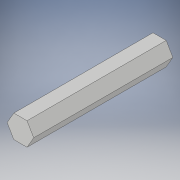
# Autodesk Inventor part: 525 hex shaft
Saved by Autodesk Inventor 2018 (Build 220112000, 112)
## iProperties
Created: 2018-07-02
Part Number: 525 hex shaft
Material: Generic
Document SubType Name: Modeling
Designer: s-2512711
Density: 1 g/cm^3
Appearance: Default
Author: s-2512711
Autodesk Inventor part; units mm, degrees
ref_plane "YZ Plane" through (0, 0, 0) normal (1, 0, 0) x (0, 1, 0)
ref_plane "XZ Plane" through (0, 0, 0) normal (0, 1, 0) x (-1, 0, 0)
ref_plane "XY Plane" through (0, 0, 0) normal (0, 0, 1) x (1, 0, 0)
sketch "Sketch1" plane through (0, 0, 0) normal (0, 0, 1) x (1, 0, 0)
  line L0 (12.7, 0) -> (6.35, -10.9985)
  line L1 (6.35, -10.9985) -> (-6.35, -10.9985)
  line L2 (-6.35, -10.9985) -> (-12.7, 0)
  line L3 (-12.7, 0) -> (-6.35, 10.9985)
  line L4 (-6.35, 10.9985) -> (6.35, 10.9985)
  line L5 (6.35, 10.9985) -> (12.7, 0)
  point P0 (0, 0)
  point P1 (0, 0)
  dimension "d0" = 12.7
  constraints: 12 end point, 1 coincident, 13 other
  measures "d0" distance of L3.end L4.end
extrude "Extrusion1" add sketch "Sketch1" along normal blind 133.35
body "Solid1"
